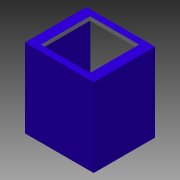
# Autodesk Inventor part: brain box bottom
Saved by Autodesk Inventor 2015 (Build 190159000, 159)
## iProperties
Created: 2014-09-09
Part Number: brain box bottom
Material: Generic
Document SubType Name: Modeling
Designer: ericd_000
Density: 1 g/cm^3
Appearance: Default
Author: ericd_000
Autodesk Inventor part; units mm, degrees
ref_plane "YZ Plane" through (0, 0, 0) normal (1, 0, 0) x (0, 1, 0)
ref_plane "XZ Plane" through (0, 0, 0) normal (0, 1, 0) x (-1, 0, 0)
ref_plane "XY Plane" through (0, 0, 0) normal (0, 0, 1) x (1, 0, 0)
sketch "Sketch1" plane through (0, 0, 0) normal (0, 1, 0) x (-1, 0, 0)
  line L0 (70, 80) -> (-70, 80)
  line L1 (-70, 80) -> (-70, -80)
  line L2 (-70, -80) -> (70, -80)
  line L3 (70, -80) -> (70, 80)
  point P0 (0, 0)
  point P1 (70, 0)
  point P2 (0, -80)
  dimension "d0" = 160
  dimension "d1" = 140
  constraints: 8 end point, 2 midpoint, 2 parallel, 1 horizontal, 1 horizontal alignment, 1 perpendicular, 1 vertical alignment
  measures "d0" distance of L2.end L0.start
  measures "d1" distance of L0.start L0.end
extrude "Extrusion1" add sketch "Sketch1" along normal blind 5
sketch "Sketch2" plane through (0, 5, 0) normal (0, 1, 0) x (1, 0, 0)
  line L0 (-70, -80) -> (70, -80)
  line L1 (70, -80) -> (70, 80)
  line L2 (70, 80) -> (-70, 80)
  line L3 (-70, 80) -> (-70, -80)
  line L4 (-62, -72) -> (62, -72)
  line L5 (62, -72) -> (62, 72)
  line L6 (62, 72) -> (-62, 72)
  line L7 (-62, 72) -> (-62, -72)
  point P0 (0, 0)
  dimension "d4" = 8
  constraints: 16 end point, 4 parallel, 2 perpendicular, 1 horizontal, 3 other
  measures "d4" distance between parallel lines of L3 L7
extrude "Extrusion2" add sketch "Sketch2" along normal blind 120
sketch "Sketch3" plane through (0, 125, 0) normal (0, 1, 0) x (1, 0, 0)
  circle A0 centre (-66, 76) radius 1.5
  circle A1 centre (66, 76) radius 1.5
  circle A2 centre (66, -76) radius 1.5
  circle A3 centre (-66, -76) radius 1.5
  line L0 (70, -80) -> (70, 80) projected
  line L1 (-70, -80) -> (70, -80) projected
  line L2 (70, 80) -> (-70, 80) projected
  line L3 (-70, 80) -> (-70, -80) projected
  point P0 (0, 0)
  dimension "d8" = 3
  dimension "d12" = 4
  dimension "d16" = 4
  dimension "d18" = 3
  dimension "d19" = 4
  dimension "d20" = 4
  dimension "d21" = 3
  dimension "d22" = 4
  dimension "d23" = 4
  dimension "d24" = 4
  dimension "d25" = 4
  dimension "d26" = 3
  constraints: 4 centre point
  measures "d8" diameter of A1
  measures "d12" distance from line of A1.centre L0
  measures "d16" distance from line of L2 A1.centre
  measures "d18" diameter of A0
  measures "d19" distance from line of L3 A0.centre
  measures "d20" distance from line of L2 A0.centre
  measures "d21" diameter of A2
  measures "d22" distance from line of L0 A2.centre
  measures "d23" distance from line of L1 A2.centre
  measures "d24" distance from line of L3 A3.centre
  measures "d25" distance from line of A3.centre L1
  measures "d26" diameter of A3
extrude "Extrusion3" cut sketch "Sketch3" against normal blind 15 contours A0 | A1 | A2 | A3
sketch "Sketch4" plane through (70, 0, 80) normal (1, 0, 0) x (0, 0, -1)
  line L0 (30, 112.5) -> (130, 112.5)
  line L1 (130, 112.5) -> (130, 12.5)
  line L2 (130, 12.5) -> (30, 12.5)
  line L3 (30, 12.5) -> (30, 112.5)
  line L4 (0, 125) -> (160, 125) projected
  line L5 (160, 0) -> (160, 125) projected
  point P0 (80, 0)
  point P1 (80, 112.5)
  point P2 (80, 125)
  point P3 (130, 62.5)
  point P4 (160, 62.5)
  dimension "d29" = 100
  dimension "d30" = 100
  constraints: 8 end point, 4 midpoint, 2 parallel, 1 horizontal, 1 horizontal alignment, 1 perpendicular, 1 vertical alignment
  measures "d29" distance of L0.start L0.end
  measures "d30" distance of L2.end L0.start
sketch "Sketch5" plane through (-70, 0, 80) normal (0, 0, 1) x (1, 0, 0)
  line L0 (20, 112.5) -> (120, 112.5)
  line L1 (120, 112.5) -> (120, 12.5)
  line L2 (120, 12.5) -> (20, 12.5)
  line L3 (20, 12.5) -> (20, 112.5)
  line L4 (140, 0) -> (140, 125) projected
  line L5 (0, 125) -> (140, 125) projected
  point P0 (70, 0)
  point P1 (120, 62.5)
  point P2 (140, 62.5)
  point P3 (70, 112.5)
  point P4 (70, 125)
  dimension "d31" = 100
  dimension "d32" = 100
  constraints: 8 end point, 4 midpoint, 2 parallel, 1 horizontal, 1 horizontal alignment, 1 perpendicular, 1 vertical alignment
  measures "d31" distance of L0.start L0.end
  measures "d32" distance of L0.end L1.end
extrude "Extrusion4" cut sketch "Sketch5" against normal blind 10
body "Solid1"
